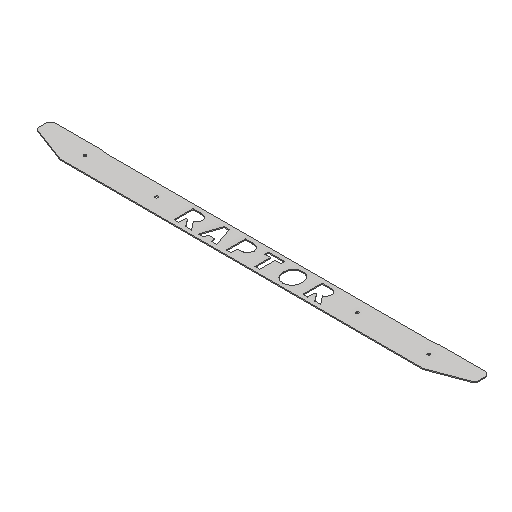
# Autodesk Inventor part: LC_ALU_1mm_Heatbed_Platform_Logo_Plate
Saved by Autodesk Inventor 2026.1 (Build 301233000, 233)
## iProperties
Created: 2016-06-27
Part Number: LC_ALU_1mm_Heatbed_Platform_Logo_Plate
Material: Ogólny
Document SubType Name: Modeling
Designer: Andrzej
Density: 1 g/cm^3
Appearance: Obrobione — aluminium
Author: Andrzej
Autodesk Inventor part; units mm, degrees
ref_plane "YZ Plane" through (0, 0, 0) normal (1, 0, 0) x (0, 1, 0)
ref_plane "XZ Plane" through (0, 0, 0) normal (0, 1, 0) x (-1, 0, 0)
ref_plane "XY Plane" through (0, 0, 0) normal (0, 0, 1) x (1, 0, 0)
sketch "Szkic1" plane through (0, 0, 0) normal (0, 0, 1) x (1, 0, 0)
  line L0 (444.72319, 18.712041) -> (444.72319, -11.287959)
  line L1 (444.72319, -11.287959) -> (-15.27681, -11.287959)
  line L2 (-15.27681, -11.287959) -> (-15.27681, 18.712041)
  line L3 (-15.27681, 18.712041) -> (36.12319, 18.712041)
  line L4 (36.12319, 18.712041) -> (36.12319, 17.712041)
  line L5 (36.12319, 17.712041) -> (393.32319, 17.712041)
  line L6 (393.32319, 17.712041) -> (393.32319, 18.712041)
  line L7 (393.32319, 18.712041) -> (444.72319, 18.712041)
  point P0 (0, 0)
  dimension "d0" = 460
  dimension "d1" = 30
  dimension "d2" = 1
  dimension "d3" = 51.4
  dimension "d4" = 51.4
  constraints: 16 end point, 4 perpendicular, 1 horizontal, 1 parallel, 1 point on line
  measures "d0" distance of L0.end L1.end
  measures "d1" distance of L0.start L0.end
  measures "d2" distance between parallel lines of L3 L5
  measures "d3" distance of L2.end L3.end
  measures "d4" distance of L6.end L0.start
extrude "Wyciągnięcie proste1" add sketch "Szkic1" along normal blind 1
chamfer "Faza1" distance 10 distance2 1 1 edges at (36.1232, 17.712, 0.5) measured on face at (274.2565, 17.712, 0.6667)
chamfer "Faza2" distance 10 distance2 1 1 edges at (393.3232, 17.712, 0.5) measured on face at (277.5898, 17.712, 0.3333)
fillet "Zaokrąglenie1" radius 5 2 edges at (444.7232, 18.712, 0.5) (-15.2768, 18.712, 0.5)
chamfer "Faza3" distance 40 distance2 15 1 edges at (444.7232, -11.288, 0.5) measured on face at (138.0565, -11.288, 0.3333)
chamfer "Faza4" distance 40 distance2 15 1 edges at (-15.2768, -11.288, 0.5) measured on face at (124.7232, -11.288, 0.3333)
sketch "Szkic2" plane through (0, 0, 1) normal (0, 0, 1) x (1, 0, 0)
  line L0 (137.22319, 13.612041) -> (416.609264, 13.612041) construction
  line L1 (416.609264, 13.612041) -> (416.609264, -7.103164) construction
  line L2 (416.609264, -7.103164) -> (137.22319, -7.103164) construction
  line L3 (137.22319, -7.103164) -> (137.22319, 13.612041) construction
  line L4 (383.32319, 17.712041) -> (46.12319, 17.712041)
  line L5 (-15.27681, 13.712041) -> (-15.27681, 3.712041)
  line L6 (444.72319, 3.712041) -> (444.72319, 13.712041)
  line L7 (24.72319, -11.287959) -> (404.72319, -11.287959)
  line L8 (24.72319, -11.287959) -> (-15.27681, 3.712041)
  line L9 (24.72319, -11.287959) -> (404.72319, -11.287959)
  line L10 (444.72319, 3.712041) -> (404.72319, -11.287959)
  line L11 (444.72319, 3.712041) -> (444.72319, 13.712041)
  arc A0 (444.72319, 13.712041) -> (439.72319, 18.712041) centre (439.72319, 13.712041) ccw
  line L12 (439.72319, 18.712041) -> (393.32319, 18.712041)
  line L13 (383.32319, 17.712041) -> (393.32319, 18.712041)
  line L14 (383.32319, 17.712041) -> (46.12319, 17.712041)
  line L15 (36.12319, 18.712041) -> (46.12319, 17.712041)
  line L16 (36.12319, 18.712041) -> (-10.27681, 18.712041)
  arc A1 (-10.27681, 18.712041) -> (-15.27681, 13.712041) centre (-10.27681, 13.712041) ccw
  line L17 (-15.27681, 13.712041) -> (-15.27681, 3.712041)
  line L18 (157.774243, -6.809352) -> (151.664033, -6.809352)
  line L19 (151.664033, -6.809352) -> (146.104875, 0.532625)
  line L20 (146.104875, 0.532625) -> (144.28964, 0.532625)
  line L21 (144.28964, 0.532625) -> (144.28964, -6.809352)
  line L22 (144.28964, -6.809352) -> (139.297744, -6.809352)
  line L23 (139.297744, -6.809352) -> (139.297744, 13.190648)
  line L24 (139.297744, 13.190648) -> (147.336642, 13.190648)
  spline S0 degree 2 poles (147.336642, 13.190648) (149.00601, 13.190648) (151.469543, 12.769254) (152.523028, 12.120956) knots 0 0 0 1 2 2 2
  spline S1 degree 2 poles (152.523028, 12.120956) (153.59272, 11.440243) (154.856901, 9.317066) (154.856901, 7.69632) knots 0 0 0 1 2 2 2
  spline S2 degree 2 poles (154.856901, 7.69632) (154.856901, 5.411069) (152.782347, 2.54235) (151.048149, 1.699562) knots 0 0 0 1 2 2 2
  line L25 (151.048149, 1.699562) -> (157.774243, -6.809352)
  spline S3 degree 2 poles (149.70293, 7.06423) (149.70293, 7.82598) (149.119462, 8.91188) (148.454956, 9.203614) knots 0 0 0 1 2 2 2
  spline S4 degree 2 poles (148.454956, 9.203614) (147.98494, 9.398103) (146.834211, 9.511555) (145.975216, 9.511555) knots 0 0 0 1 2 2 2
  line L26 (145.975216, 9.511555) -> (144.28964, 9.511555)
  line L27 (144.28964, 9.511555) -> (144.28964, 4.13068)
  line L28 (144.28964, 4.13068) -> (145.732104, 4.13068)
  spline S5 degree 2 poles (145.732104, 4.13068) (146.769381, 4.13068) (148.244259, 4.39) (148.746691, 4.795186) knots 0 0 0 1 2 2 2
  spline S6 degree 2 poles (148.746691, 4.795186) (149.232914, 5.184165) (149.70293, 6.221442) (149.70293, 7.06423) knots 0 0 0 1 2 2 2
  line L29 (165.164843, -6.809352) -> (171.923352, 13.190648)
  line L30 (171.923352, 13.190648) -> (177.401472, 13.190648)
  line L31 (177.401472, 13.190648) -> (184.159981, -6.809352)
  line L32 (184.159981, -6.809352) -> (178.989802, -6.809352)
  line L33 (178.989802, -6.809352) -> (177.741828, -2.725073)
  line L34 (177.741828, -2.725073) -> (171.453336, -2.725073)
  line L35 (171.453336, -2.725073) -> (170.189154, -6.809352)
  line L36 (170.189154, -6.809352) -> (165.164843, -6.809352)
  line L37 (176.639721, 0.905397) -> (174.597582, 7.518038)
  line L38 (174.597582, 7.518038) -> (172.539235, 0.905397)
  line L39 (172.539235, 0.905397) -> (176.639721, 0.905397)
  spline S7 degree 2 poles (209.589478, 6.885948) (209.589478, 5.492106) (208.698068, 2.963743) (207.871488, 2.120956) knots 0 0 0 1 2 2 2
  spline S8 degree 2 poles (207.871488, 2.120956) (207.369057, 1.58611) (206.13729, 0.710907) (205.407955, 0.402965) knots 0 0 0 1 2 2 2
  spline S9 degree 2 poles (205.407955, 0.402965) (204.662412, 0.095024) (202.928214, -0.26154) (201.858522, -0.26154) knots 0 0 0 1 2 2 2
  line L40 (201.858522, -0.26154) -> (199.232914, -0.26154)
  line L41 (199.232914, -0.26154) -> (199.232914, -6.809352)
  line L42 (199.232914, -6.809352) -> (194.208603, -6.809352)
  line L43 (194.208603, -6.809352) -> (194.208603, 13.190648)
  line L44 (194.208603, 13.190648) -> (201.971974, 13.190648)
  spline S10 degree 2 poles (201.971974, 13.190648) (203.689964, 13.190648) (206.20212, 12.558557) (207.22319, 11.877844) knots 0 0 0 1 2 2 2
  spline S11 degree 2 poles (207.22319, 11.877844) (208.357712, 11.116094) (209.589478, 8.620145) (209.589478, 6.885948) knots 0 0 0 1 2 2 2
  spline S12 degree 2 poles (204.435507, 6.756288) (204.435507, 7.615283) (203.625135, 8.830842) (203.074081, 9.057747) knots 0 0 0 1 2 2 2
  spline S13 degree 2 poles (203.074081, 9.057747) (202.360953, 9.365688) (201.064357, 9.462933) (199.946042, 9.462933) knots 0 0 0 1 2 2 2
  line L45 (199.946042, 9.462933) -> (199.232914, 9.462933)
  line L46 (199.232914, 9.462933) -> (199.232914, 3.466175)
  line L47 (199.232914, 3.466175) -> (199.589478, 3.466175)
  spline S14 degree 2 poles (199.589478, 3.466175) (200.286399, 3.466175) (201.55058, 3.498589) (202.020597, 3.579627) knots 0 0 0 1 2 2 2
  spline S15 degree 2 poles (202.020597, 3.579627) (202.425783, 3.644457) (203.317193, 4.033435) (203.560305, 4.276547) knots 0 0 0 1 2 2 2
  spline S16 degree 2 poles (203.560305, 4.276547) (204.078943, 4.762771) (204.435507, 5.848671) (204.435507, 6.756288) knots 0 0 0 1 2 2 2
  line L48 (224.176188, -6.809352) -> (224.176188, 9.381896)
  line L49 (224.176188, 9.381896) -> (218.260467, 9.381896)
  line L50 (218.260467, 9.381896) -> (218.260467, 13.190648)
  line L51 (218.260467, 13.190648) -> (235.116221, 13.190648)
  line L52 (235.116221, 13.190648) -> (235.116221, 9.381896)
  line L53 (235.116221, 9.381896) -> (229.200499, 9.381896)
  line L54 (229.200499, 9.381896) -> (229.200499, -6.809352)
  line L55 (229.200499, -6.809352) -> (224.176188, -6.809352)
  spline S17 degree 2 poles (263.430645, 3.190648) (263.430645, -1.671589) (258.244259, -7.230746) (253.738587, -7.230746) knots 0 0 0 1 2 2 2
  spline S18 degree 2 poles (253.738587, -7.230746) (249.216707, -7.230746) (244.062736, -1.606759) (244.062736, 3.190648) knots 0 0 0 1 2 2 2
  spline S19 degree 2 poles (244.062736, 3.190648) (244.062736, 8.004262) (249.216707, 13.612042) (253.738587, 13.612042) knots 0 0 0 1 2 2 2
  spline S20 degree 2 poles (253.738587, 13.612042) (258.244259, 13.612042) (263.430645, 8.036677) (263.430645, 3.190648) knots 0 0 0 1 2 2 2
  spline S21 degree 2 poles (258.244259, 3.190648) (258.244259, 4.989675) (257.514924, 7.501831) (256.882833, 8.295996) knots 0 0 0 1 2 2 2
  spline S22 degree 2 poles (256.882833, 8.295996) (256.250742, 9.122577) (254.629997, 9.835705) (253.754794, 9.835705) knots 0 0 0 1 2 2 2
  spline S23 degree 2 poles (253.754794, 9.835705) (252.830969, 9.835705) (251.323676, 9.171199) (250.626755, 8.328411) knots 0 0 0 1 2 2 2
  spline S24 degree 2 poles (250.626755, 8.328411) (250.010872, 7.550453) (249.249122, 4.973468) (249.249122, 3.190648) knots 0 0 0 1 2 2 2
  spline S25 degree 2 poles (249.249122, 3.190648) (249.249122, 1.342998) (249.978457, -1.08812) (250.610548, -1.914701) knots 0 0 0 1 2 2 2
  spline S26 degree 2 poles (250.610548, -1.914701) (251.242639, -2.741281) (252.879592, -3.454409) (253.754794, -3.454409) knots 0 0 0 1 2 2 2
  spline S27 degree 2 poles (253.754794, -3.454409) (254.646204, -3.454409) (256.299365, -2.692659) (256.899041, -1.882286) knots 0 0 0 1 2 2 2
  spline S28 degree 2 poles (256.899041, -1.882286) (257.547339, -1.007083) (258.244259, 1.310583) (258.244259, 3.190648) knots 0 0 0 1 2 2 2
  line L56 (292.944422, -6.809352) -> (286.834211, -6.809352)
  line L57 (286.834211, -6.809352) -> (281.275054, 0.532625)
  line L58 (281.275054, 0.532625) -> (279.459819, 0.532625)
  line L59 (279.459819, 0.532625) -> (279.459819, -6.809352)
  line L60 (279.459819, -6.809352) -> (274.467922, -6.809352)
  line L61 (274.467922, -6.809352) -> (274.467922, 13.190648)
  line L62 (274.467922, 13.190648) -> (282.50682, 13.190648)
  spline S29 degree 2 poles (282.50682, 13.190648) (284.176188, 13.190648) (286.639721, 12.769254) (287.693206, 12.120956) knots 0 0 0 1 2 2 2
  spline S30 degree 2 poles (287.693206, 12.120956) (288.762898, 11.440243) (290.02708, 9.317066) (290.02708, 7.69632) knots 0 0 0 1 2 2 2
  spline S31 degree 2 poles (290.02708, 7.69632) (290.02708, 5.411069) (287.952525, 2.54235) (286.218328, 1.699562) knots 0 0 0 1 2 2 2
  line L63 (286.218328, 1.699562) -> (292.944422, -6.809352)
  spline S32 degree 2 poles (284.873109, 7.06423) (284.873109, 7.82598) (284.28964, 8.91188) (283.625135, 9.203614) knots 0 0 0 1 2 2 2
  spline S33 degree 2 poles (283.625135, 9.203614) (283.155118, 9.398103) (282.004389, 9.511555) (281.145394, 9.511555) knots 0 0 0 1 2 2 2
  line L64 (281.145394, 9.511555) -> (279.459819, 9.511555)
  line L65 (279.459819, 9.511555) -> (279.459819, 4.13068)
  line L66 (279.459819, 4.13068) -> (280.902282, 4.13068)
  spline S34 degree 2 poles (280.902282, 4.13068) (281.939559, 4.13068) (283.414438, 4.39) (283.916869, 4.795186) knots 0 0 0 1 2 2 2
  spline S35 degree 2 poles (283.916869, 4.795186) (284.403093, 5.184165) (284.873109, 6.221442) (284.873109, 7.06423) knots 0 0 0 1 2 2 2
  point P0 (0, 0)
  point P1 (34.72319, 4.712041)
  point P2 (394.72319, 4.712041)
  point P3 (109.72319, 4.712041)
  point P4 (319.72319, 4.712041)
  dimension "d34" = 50
  dimension "d35" = 75
  dimension "d36" = 75
  dimension "d37" = 50
  dimension "d38" = 152.5
  dimension "d42" = 4.1
  dimension "d43" = 14
  dimension "d44" = 14
  dimension "d45" = 14
  dimension "d46" = 14
  constraints: 2 other
  measures "d34" distance from line of point (34.723, 4.712) L5
  measures "d35" distance of point (34.723, 4.712) point (109.723, 4.712)
  measures "d36" distance of point (394.723, 4.712) point (319.723, 4.712)
  measures "d37" distance from line of L6 point (394.723, 4.712)
  measures "d38" distance between parallel lines of L5 L3
  measures "d42" distance between parallel lines of L4 L0
  measures "d43" distance from line of L16 point (34.723, 4.712)
  measures "d44" distance from line of L16 point (109.723, 4.712)
  measures "d45" distance from line of L12 point (319.723, 4.712)
  measures "d46" distance from line of L12 point (394.723, 4.712)
extrude "Wyciągnięcie proste2" cut sketch "Szkic2" against normal blind 5 contours L18 L19 L20 L21 L22 L23 L24 S0 S1 S2 L25 | L29 L30 L31 L32 L33 L34 L35 L36 | S7 S8 S9 L40 L41 L42 L43 L44 S10 S11 | L48 L49 L50 L51 L52 L53 L54 L55 | S17 S18 S19 S20 | L56 L57 L58 L59 L60 L61 L62 S29 S30 S31 L63
fillet "Zaokrąglenie2" radius 3 4 edges at (444.7232, 3.712, 0.5) (404.7232, -11.288, 0.5) (24.7232, -11.288, 0.5) (-15.2768, 3.712, 0.5)
hole "Otwór1" at (34.72319, 4.712041, 1) at (394.72319, 4.712041, 1) at (109.72319, 4.712041, 1) at (319.72319, 4.712041, 1) direction (0, 0, -1) diameter 3 end through all
sketch "Szkic4" plane through (0, 0, 1) normal (0, 0, 1) x (1, 0, 0)
  circle A0 centre (109.72319, 4.712041) radius 1.5
  circle A1 centre (34.72319, 4.712041) radius 1.5
  circle A2 centre (394.72319, 4.712041) radius 1.5
  circle A3 centre (319.72319, 4.712041) radius 1.5
  arc A4 (-15.27681, 5.791042) -> (-13.330181, 2.982055) centre (-12.27681, 5.791042) ccw
  line L0 (24.213823, -11.096947) -> (-13.330181, 2.982055)
  arc A5 (24.213823, -11.096947) -> (25.267193, -11.287959) centre (25.267193, -8.287959) ccw
  line L1 (25.267193, -11.287959) -> (404.179186, -11.287959)
  arc A6 (404.179186, -11.287959) -> (405.232556, -11.096947) centre (404.179186, -8.287959) ccw
  line L2 (442.77656, 2.982055) -> (405.232556, -11.096947)
  arc A7 (442.77656, 2.982055) -> (444.72319, 5.791042) centre (441.72319, 5.791042) ccw
  line L3 (444.72319, 5.791042) -> (444.72319, 13.712041)
  arc A8 (444.72319, 13.712041) -> (439.72319, 18.712041) centre (439.72319, 13.712041) ccw
  line L4 (439.72319, 18.712041) -> (393.32319, 18.712041)
  line L5 (383.32319, 17.712041) -> (393.32319, 18.712041)
  line L6 (383.32319, 17.712041) -> (46.12319, 17.712041)
  line L7 (36.12319, 18.712041) -> (46.12319, 17.712041)
  line L8 (36.12319, 18.712041) -> (-10.27681, 18.712041)
  arc A9 (-10.27681, 18.712041) -> (-15.27681, 13.712041) centre (-10.27681, 13.712041) ccw
  line L9 (-15.27681, 13.712041) -> (-15.27681, 5.791042)
  line L10 (286.218328, 1.699562) -> (292.944422, -6.809352)
  line L11 (292.944422, -6.809352) -> (286.834211, -6.809352)
  line L12 (286.834211, -6.809352) -> (281.275054, 0.532625)
  line L13 (281.275054, 0.532625) -> (279.459819, 0.532625)
  line L14 (279.459819, 0.532625) -> (279.459819, -6.809352)
  line L15 (279.459819, -6.809352) -> (274.467922, -6.809352)
  line L16 (274.467922, -6.809352) -> (274.467922, 13.190648)
  line L17 (274.467922, 13.190648) -> (282.50682, 13.190648)
  line L18 (171.453336, -2.725073) -> (170.189154, -6.809352)
  line L19 (157.774243, -6.809352) -> (151.664033, -6.809352)
  line L20 (151.664033, -6.809352) -> (146.104875, 0.532625)
  line L21 (146.104875, 0.532625) -> (144.28964, 0.532625)
  line L22 (144.28964, 0.532625) -> (144.28964, -6.809352)
  line L23 (144.28964, -6.809352) -> (139.297744, -6.809352)
  line L24 (139.297744, -6.809352) -> (139.297744, 13.190648)
  line L25 (139.297744, 13.190648) -> (147.336642, 13.190648)
  line L26 (151.048149, 1.699562) -> (157.774243, -6.809352)
  line L27 (165.164843, -6.809352) -> (171.923352, 13.190648)
  line L28 (171.923352, 13.190648) -> (177.401472, 13.190648)
  line L29 (177.401472, 13.190648) -> (184.159981, -6.809352)
  line L30 (184.159981, -6.809352) -> (178.989802, -6.809352)
  line L31 (178.989802, -6.809352) -> (177.741828, -2.725073)
  line L32 (177.741828, -2.725073) -> (171.453336, -2.725073)
  line L33 (201.858522, -0.26154) -> (199.232914, -0.26154)
  line L34 (199.232914, -0.26154) -> (199.232914, -6.809352)
  line L35 (199.232914, -6.809352) -> (194.208603, -6.809352)
  line L36 (194.208603, -6.809352) -> (194.208603, 13.190648)
  line L37 (194.208603, 13.190648) -> (201.971974, 13.190648)
  line L38 (229.200499, -6.809352) -> (224.176188, -6.809352)
  line L39 (224.176188, -6.809352) -> (224.176188, 9.381896)
  line L40 (224.176188, 9.381896) -> (218.260467, 9.381896)
  line L41 (218.260467, 9.381896) -> (218.260467, 13.190648)
  line L42 (218.260467, 13.190648) -> (235.116221, 13.190648)
  line L43 (235.116221, 13.190648) -> (235.116221, 9.381896)
  line L44 (235.116221, 9.381896) -> (229.200499, 9.381896)
  line L45 (229.200499, 9.381896) -> (229.200499, -6.809352)
  spline S0 degree 2 poles (148.454956, 9.203614) (147.98494, 9.398103) (146.834211, 9.511555) (145.975216, 9.511555) knots 0 0 0 0.5 1 1 1
  line L46 (145.975216, 9.511555) -> (144.28964, 9.511555)
  line L47 (144.28964, 9.511555) -> (144.28964, 4.13068)
  line L48 (144.28964, 4.13068) -> (145.732104, 4.13068)
  spline S1 degree 2 poles (145.732104, 4.13068) (146.769381, 4.13068) (148.244259, 4.39) (148.747469, 4.794217) (148.747469, 4.794217) knots 0 0 0 0.49999999 0.99999998 1 1 1
  spline S2 degree 2 poles (148.746691, 4.795186) (149.232914, 5.184165) (149.70293, 6.221442) (149.70293, 7.06423) knots 0 0 0 0.5 1 1 1
  spline S3 degree 2 poles (149.70293, 7.06423) (149.70293, 7.82598) (149.119462, 8.91188) (148.454956, 9.203614) knots 0 0 0 0.5 1 1 1
  line L49 (174.597582, 7.518038) -> (172.539235, 0.905397)
  line L50 (172.539235, 0.905397) -> (176.639721, 0.905397)
  line L51 (176.639721, 0.905397) -> (174.597582, 7.518038)
  spline S4 degree 2 poles (203.074081, 9.057747) (202.360953, 9.365688) (201.064357, 9.462933) (199.946042, 9.462933) knots 0 0 0 0.5 1 1 1
  line L52 (199.946042, 9.462933) -> (199.232914, 9.462933)
  line L53 (199.232914, 9.462933) -> (199.232914, 3.466175)
  spline S5 degree 2 poles (203.560305, 4.276547) (204.078943, 4.762771) (204.435507, 5.848671) (204.435507, 6.756288) knots 0 0 0 0.5 1 1 1
  spline S6 degree 2 poles (204.435507, 6.756288) (204.435507, 7.615283) (203.625135, 8.830842) (203.074081, 9.057747) knots 0 0 0 0.5 1 1 1
  spline S7 degree 2 poles (256.882833, 8.295996) (256.250742, 9.122577) (254.629997, 9.835705) (253.754794, 9.835705) knots 0 0 0 0.5 1 1 1
  spline S8 degree 2 poles (253.754794, 9.835705) (252.830969, 9.835705) (251.323676, 9.171199) (250.626755, 8.328411) knots 0 0 0 0.5 1 1 1
  spline S9 degree 2 poles (250.626755, 8.328411) (250.010872, 7.550453) (249.249122, 4.973468) (249.249122, 3.190648) knots 0 0 0 0.5 1 1 1
  spline S10 degree 2 poles (249.249122, 3.190648) (249.249122, 1.342998) (249.978457, -1.08812) (250.610548, -1.914701) knots 0 0 0 0.5 1 1 1
  spline S11 degree 2 poles (250.610548, -1.914701) (251.242639, -2.741281) (252.879592, -3.454409) (253.754794, -3.454409) knots 0 0 0 0.5 1 1 1
  spline S12 degree 2 poles (253.754794, -3.454409) (254.646204, -3.454409) (256.299365, -2.692659) (256.899242, -1.882435) knots 0 0 0 0.5 1 1 1
  spline S13 degree 2 poles (256.899041, -1.882286) (257.547339, -1.007083) (258.244259, 1.310583) (258.244259, 3.190648) knots 0 0 0 0.5 1 1 1
  spline S14 degree 2 poles (258.244259, 3.190648) (258.244259, 4.989675) (257.514924, 7.501831) (256.882833, 8.295996) knots 0 0 0 0.5 1 1 1
  spline S15 degree 2 poles (283.625135, 9.203614) (283.155118, 9.398103) (282.004389, 9.511555) (281.145394, 9.511555) knots 0 0 0 0.5 1 1 1
  line L54 (281.145394, 9.511555) -> (279.459819, 9.511555)
  line L55 (279.459819, 9.511555) -> (279.459819, 4.13068)
  line L56 (279.459819, 4.13068) -> (280.902282, 4.13068)
  spline S16 degree 2 poles (280.902282, 4.13068) (281.939559, 4.13068) (283.414438, 4.39) (283.917647, 4.794217) (283.917647, 4.794217) knots 0 0 0 0.49999999 0.99999998 1 1 1
  spline S17 degree 2 poles (283.916869, 4.795186) (284.403093, 5.184165) (284.873109, 6.221442) (284.873109, 7.06423) knots 0 0 0 0.5 1 1 1
  spline S18 degree 2 poles (284.873109, 7.06423) (284.873109, 7.82598) (284.28964, 8.91188) (283.625135, 9.203614) knots 0 0 0 0.5 1 1 1
  line L57 (170.189154, -6.809352) -> (165.164843, -6.809352)
  line L58 (199.232914, 3.466175) -> (199.589478, 3.466175)
  spline S19 degree 2 poles (199.589478, 3.466175) (200.286399, 3.466175) (201.55058, 3.498589) (202.020597, 3.579627) knots 0 0 0 0.5 1 1 1
  spline S20 degree 2 poles (202.020597, 3.579627) (202.425783, 3.644457) (203.317193, 4.033435) (203.560305, 4.276547) knots 0 0 0 0.5 1 1 1
  point P0 (0, 0)
  constraints: 36 other
extrude "Wyciągnięcie proste3" cut sketch "Szkic4" against normal through all contours S3 S2 S1 L48 L47 L46 S0 | L51 L50 L49 | S6 S5 S20 S19 L58 L53 L52 S4 | S14 S13 S12 S11 S10 S9 S8 S7 | S18 S17 S16 L56 L55 L54 S15
equation "\"d4\" = d3"
equation "\"d37\" = d34"
equation "\"d44\" = d43"
equation "\"d45\" = d43"
equation "\"d46\" = d43"
